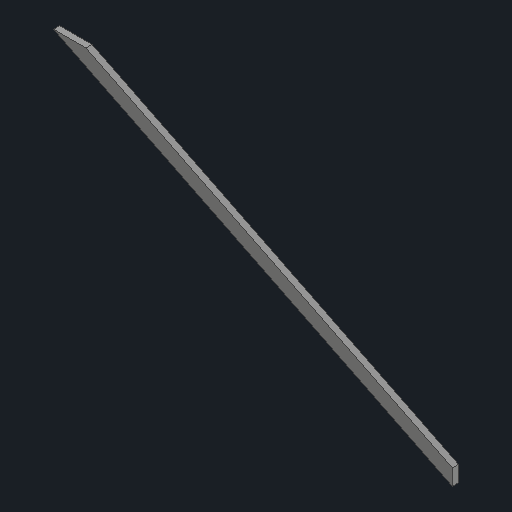
# Autodesk Inventor part: S_2x4x108.675
Saved by Autodesk Inventor 2026 (Build 300175000, 175)
## iProperties
Created: 2024-09-19
Part Number: S_2x4x108.675
Material: Generic
Document SubType Name: Modeling
Designer: User
Density: 1 g/cm^3
Appearance: Default
Author: User
Autodesk Inventor part; units mm, degrees
ref_plane "YZ Plane" through (0, 0, 0) normal (1, 0, 0) x (0, 1, 0)
ref_plane "XZ Plane" through (0, 0, 0) normal (0, 1, 0) x (-1, 0, 0)
ref_plane "XY Plane" through (0, 0, 0) normal (0, 0, 1) x (1, 0, 0)
sketch "Sketch1" plane through (0, 0, 0) normal (0, 0, 1) x (1, 0, 0)
  line L0 (0, -609.6) -> (-2438.4, -609.6) projected
  line L1 (0, -1828.8) -> (0, 1828.8) projected
  line L2 (-2476.5, -609.6) -> (-2438.4, -609.6) projected
  line L3 (-2476.5, -609.6) -> (0, -1828.8)
  line L4 (-2476.5, -609.6) -> (-2275.2249, -609.6)
  line L5 (-2275.2249, -609.6) -> (0, -1729.7107)
  line L6 (0, -1729.7107) -> (0, -1828.8)
  point P0 (0, 0)
  dimension "d0" = 88.9
  constraints: 8 end point, 2 point on line, 1 collinear, 1 parallel, 2 other
  measures "d0" distance between parallel lines of L5 L3
extrude "Extrusion1" add sketch "Sketch1" against normal blind 38.1 contours L5 L1 L3 L2 L0
body "Solid1"
